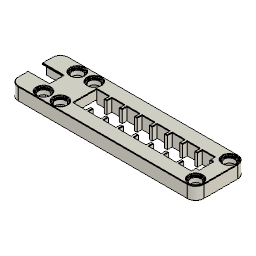
Mltplxr Chassis (Autodesk Fusion 360 design; units mm, degrees)
Autodesk Fusion 360 part; units mm, degrees
sketch "Skizze1" plane through (0, 0, 0) normal (0, 0, 1) x (1, 0, 0)
  line L0 (-39.6596, 9.8) -> (41.2404, 9.8)
  line L1 (41.2404, 9.8) -> (41.2404, -10.6)
  line L2 (41.2404, -10.6) -> (-39.6596, -10.6)
  line L3 (-39.6596, -10.6) -> (-39.6596, 9.8)
  line L4 (-39.6596, 4.85) -> (-29.1596, 4.85)
  line L5 (-29.1596, 4.85) -> (-29.1596, -5.65)
  line L6 (-29.1596, -5.65) -> (-39.6596, -5.65)
  line L7 (-39.6596, -5.65) -> (-39.6596, 4.85)
  line L8 (33.2404, 5.1) -> (39.0404, 5.1)
  line L9 (39.0404, 5.1) -> (39.0404, -5.9)
  line L10 (39.0404, -5.9) -> (33.2404, -5.9)
  line L11 (33.2404, -5.9) -> (33.2404, 5.1)
  line L12 (31.8975, 5.1) -> (31.8975, -5.9)
  line L13 (31.8975, -5.9) -> (26.0975, -5.9)
  line L14 (26.0975, 5.1) -> (31.8975, 5.1)
  line L15 (26.0975, -5.9) -> (26.0975, 5.1)
  line L16 (24.7547, 5.1) -> (24.7547, -5.9)
  line L17 (24.7547, -5.9) -> (18.9547, -5.9)
  line L18 (18.9547, 5.1) -> (24.7547, 5.1)
  line L19 (18.9547, -5.9) -> (18.9547, 5.1)
  line L20 (17.6118, 5.1) -> (17.6118, -5.9)
  line L21 (17.6118, -5.9) -> (11.8118, -5.9)
  line L22 (11.8118, 5.1) -> (17.6118, 5.1)
  line L23 (11.8118, -5.9) -> (11.8118, 5.1)
  line L24 (10.469, 5.1) -> (10.469, -5.9)
  line L25 (10.469, -5.9) -> (4.669, -5.9)
  line L26 (4.669, 5.1) -> (10.469, 5.1)
  line L27 (4.669, -5.9) -> (4.669, 5.1)
  line L28 (3.3261, 5.1) -> (3.3261, -5.9)
  line L29 (3.3261, -5.9) -> (-2.4739, -5.9)
  line L30 (-2.4739, 5.1) -> (3.3261, 5.1)
  line L31 (-2.4739, -5.9) -> (-2.4739, 5.1)
  line L32 (-3.8167, 5.1) -> (-3.8167, -5.9)
  line L33 (-3.8167, -5.9) -> (-9.6167, -5.9)
  line L34 (-9.6167, 5.1) -> (-3.8167, 5.1)
  line L35 (-9.6167, -5.9) -> (-9.6167, 5.1)
  line L36 (-10.9596, 5.1) -> (-10.9596, -5.9)
  line L37 (-10.9596, -5.9) -> (-16.7596, -5.9)
  line L38 (-16.7596, 5.1) -> (-10.9596, 5.1)
  line L39 (-16.7596, -5.9) -> (-16.7596, 5.1)
  line L40 (39.0404, 2.85) -> (40.5404, 2.85)
  line L41 (40.5404, 2.85) -> (40.5404, -3.65)
  line L42 (40.5404, -3.65) -> (39.0404, -3.65)
  line L43 (31.8975, 2.85) -> (33.3975, 2.85)
  line L44 (33.3975, -3.65) -> (31.8975, -3.65)
  line L45 (24.7547, 2.85) -> (26.2547, 2.85)
  line L46 (26.2547, -3.65) -> (24.7547, -3.65)
  line L47 (17.6118, 2.85) -> (19.1118, 2.85)
  line L48 (19.1118, -3.65) -> (17.6118, -3.65)
  line L49 (10.469, 2.85) -> (11.969, 2.85)
  line L50 (11.969, -3.65) -> (10.469, -3.65)
  line L51 (3.3261, 2.85) -> (4.8261, 2.85)
  line L52 (4.8261, -3.65) -> (3.3261, -3.65)
  line L53 (-3.8167, 2.85) -> (-2.3167, 2.85)
  line L54 (-2.3167, -3.65) -> (-3.8167, -3.65)
  line L55 (-10.9596, 2.85) -> (-9.4596, 2.85)
  line L56 (-9.4596, -3.65) -> (-10.9596, -3.65)
  line L57 (-39.6596, 2.85) -> (-30.2596, 2.85)
  line L58 (-30.2596, 2.85) -> (-30.2596, -3.65)
  line L59 (-30.2596, -3.65) -> (-39.6596, -3.65)
  arc A0 (-11.4096, 9.8) -> (-6.9096, 9.8) centre (-9.1596, 9.8) ccw
  arc A1 (-30.8596, 9.8) -> (-28.8596, 9.8) centre (-29.8596, 9.8) ccw
  arc A2 (9.0404, 9.8) -> (11.0404, 9.8) centre (10.0404, 9.8) ccw
  arc A3 (28.8404, 9.8) -> (32.8404, 9.8) centre (30.8404, 9.8) ccw
  line L60 (53, -0.4) -> (55.6063, -0.4)
  arc A4 (-28.8596, -10.6) -> (-30.8596, -10.6) centre (-29.8596, -10.6) ccw
  arc A5 (-6.9096, -10.6) -> (-11.4096, -10.6) centre (-9.1596, -10.6) ccw
  arc A6 (11.0404, -10.6) -> (9.0404, -10.6) centre (10.0404, -10.6) ccw
  arc A7 (32.8404, -10.6) -> (28.8404, -10.6) centre (30.8404, -10.6) ccw
  circle A8 centre (41.2404, -0.4) radius 1
  arc A9 (41.2404, -2.4) -> (41.2404, 1.6) centre (41.2404, -0.4) ccw
  line L61 (-29.1596, 8.8) -> (-16.7596, 8.8)
  line L62 (-16.7596, 8.8) -> (-16.7596, -9.6)
  line L63 (-16.7596, -9.6) -> (-29.1596, -9.6)
  line L64 (-29.1596, -9.6) -> (-29.1596, 8.8)
  dimension "d3" = -50
  dimension "d4" = 0
  dimension "d6" = 11
  dimension "d9" = 10.5
  dimension "d10" = 5.8
  dimension "d11" = 1.3429
  dimension "d71" = 6.5
  dimension "d72" = 2.25
  dimension "d73" = 2.25
  dimension "d88" = 6.5
  dimension "d89" = 9.4
  dimension "d93" = 10.5
  dimension "d112" = 2
  dimension "d113" = 4.5
  dimension "d116" = 2
  dimension "d120" = 4
  dimension "d128" = 20.4
  dimension "d130" = 10.2
  dimension "d131" = 20.4
  dimension "d132" = 20.4
  dimension "d133" = 20.4
  dimension "d134" = 20.4
  dimension "d135" = 4.7
  dimension "d136" = 4.7
  dimension "d146" = 4.95
  dimension "d147" = 4.95
  dimension "d148" = 6.95
  dimension "d149" = 6.95
  dimension "d151" = 1.5
  dimension "d152" = 2.2
  dimension "d198" = 4
  dimension "d199" = 2
  dimension "d204" = 1
  dimension "d205" = 1
  dimension "d214" = 9.8
  dimension "d229" = 80.9
  constraint horizontal L0
  constraint vertical L1
  constraint horizontal L2
  constraint vertical L3
  constraint horizontal L4
  constraint vertical L5
  constraint horizontal L6
  constraint vertical L7
  constraint horizontal L8
  constraint vertical L9
  constraint horizontal L10
  constraint vertical L11
  constraint coincident L9 L40.start
  constraint perpendicular L9 L40
  constraint perpendicular L40 L41
  constraint coincident L9 L42.end
  constraint perpendicular L9 L42
  constraint coincident L3 L57.start
  constraint coincident L7 L57.start
  constraint perpendicular L7 L57
  constraint perpendicular L56 L58
  constraint coincident L7 L59.end
  constraint coincident L0 A0.end
  constraint coincident L0 A0.start
  constraint coincident L0 A1.end
  constraint coincident L0 A1.start
  constraint coincident L0 A2.end
  constraint coincident L0 A2.start
  constraint coincident L0 A3.end
  constraint coincident L0 A3.start
  constraint perpendicular L1 L60
  constraint symmetric A0.end L60 A5.start
  constraint symmetric A0.start L60 A5.end
  constraint symmetric A0 L60 A5
  constraint symmetric A1.end L60 A4.start
  constraint symmetric A1.start L60 A4.end
  constraint symmetric A1 L60 A4
  constraint symmetric A2.end L60 A6.start
  constraint symmetric A2.start L60 A6.end
  constraint symmetric A2 L60 A6
  constraint symmetric A3.end L60 A7.start
  constraint symmetric A3.start L60 A7.end
  constraint symmetric A3 L60 A7
  constraint horizontal L59
  constraint midpoint L1 A8.centre
  constraint concentric A8 A9
  constraint coincident L1 A9.end
  constraint coincident L1 A9.start
  constraint horizontal L61
  constraint vertical L62
  constraint horizontal L63
  constraint vertical L64
  measures "d6" distance of L8 L10
  measures "d9" distance of L4 L6
  measures "d10" distance of L9 L11
  measures "d11" distance of L11 L12
  measures "d71" distance of L40.end L41.end
  measures "d72" distance of L8 L40
  measures "d73" distance of L10 L42
  measures "d88" distance of L57.end L58.end
  measures "d89" distance of L57.start L57.end
  measures "d93" distance of L4.start L4.end
  measures "d112" diameter of A1
  measures "d113" diameter of A0
  measures "d116" diameter of A2
  measures "d120" diameter of A3
  measures "d128" distance of L0 L2
  measures "d130" distance of L2 L60
  measures "d131" distance of L2 A1.centre
  measures "d132" distance of L2 A0.centre
  measures "d133" distance of L2 A2.centre
  measures "d134" distance of L2 A3.centre
  measures "d135" distance of L0 L18
  measures "d136" distance of L2 L13
  measures "d146" distance of L0 L4
  measures "d147" distance of L2 L6
  measures "d148" distance of L0 L57
  measures "d149" distance of L2 L59
  measures "d151" distance of L9 L41
  measures "d152" distance of L1 L9
  measures "d198" diameter of A9
  measures "d199" diameter of A8
  measures "d204" distance of L0 L61
  measures "d205" distance of L2 L63
  measures "d214" distance of L0.start A1.centre
  measures "d229" distance of L1.end L2.end
sketch "Skizze2" plane through (0, 0, 0) normal (0, 0, 1) x (1, 0, 0)
  line L0 (-36.4596, 11.6) -> (43.5404, 11.6)
  line L1 (47.5404, 7.6) -> (47.5404, -8.4)
  line L2 (43.5404, -12.4) -> (-36.4596, -12.4)
  line L3 (-40.4596, -8.4) -> (-40.4596, 7.6)
  line L4 (-39.6596, 9.8) -> (41.2404, 9.8)
  line L5 (41.2404, -10.6) -> (-39.6596, -10.6)
  line L6 (-39.6596, -10.6) -> (-39.6596, 9.8)
  line L7 (39.0404, 5.1) -> (39.0404, -5.9)
  line L8 (33.2404, -5.9) -> (33.2404, 5.1)
  line L9 (-27.8596, 4) -> (-27.8596, -4.8)
  line L10 (-29.9596, -4.8) -> (-27.8596, -4.8)
  line L11 (41.2404, 9.8) -> (41.2404, -10.6)
  line L12 (-39.6596, 4.85) -> (-40.4596, 4.85)
  line L13 (-39.6596, -5.65) -> (-40.4596, -5.65)
  line L14 (-39.6596, 2.85) -> (-30.2596, 2.85)
  line L15 (-30.2596, 2.85) -> (-30.2596, -3.65)
  line L16 (-30.2596, -3.65) -> (-39.6596, -3.65)
  line L17 (-39.6596, 2.85) -> (-40.4596, 2.85)
  line L18 (-39.6596, -3.65) -> (-40.4596, -3.65)
  arc A0 (47.5404, 7.6) -> (43.5404, 11.6) centre (43.5404, 7.6) ccw
  arc A1 (43.5404, -12.4) -> (47.5404, -8.4) centre (43.5404, -8.4) ccw
  line L19 (-16.7596, -5.9) -> (-16.7596, 5.1)
  arc A2 (-6.9096, -10.6) -> (-11.4096, -10.6) centre (-9.1596, -10.6) ccw
  arc A3 (-11.4096, 9.8) -> (-6.9096, 9.8) centre (-9.1596, 9.8) ccw
  arc A4 (28.8404, 9.8) -> (32.8404, 9.8) centre (30.8404, 9.8) ccw
  arc A5 (32.8404, -10.6) -> (28.8404, -10.6) centre (30.8404, -10.6) ccw
  circle A6 centre (-9.1596, 9.1) radius 2
  line L20 (-27.8596, 4) -> (-32, 4)
  line L21 (-32, 4) -> (-32, -4.8)
  line L22 (-29.9596, -4.8) -> (-32, -4.8)
  circle A7 centre (-9.1596, 9.1) radius 0.75
  line L23 (-15.2596, 4) -> (37.5404, 4)
  line L24 (37.5404, 4) -> (37.5404, -4.8)
  line L25 (37.5404, -4.8) -> (-15.2596, -4.8)
  line L26 (-15.2596, -4.8) -> (-15.2596, 4)
  line L27 (-29.1596, -5.65) -> (-39.6596, -5.65)
  line L28 (-39.6596, 4.85) -> (-29.1596, 4.85)
  circle A8 centre (-9.1596, 9.1) radius 1.25
  line L29 (-29.1596, -5.65) -> (-30.2596, -5.65)
  line L30 (-30.2596, -5.65) -> (-30.2596, 4.85)
  line L31 (-30.2596, 4.85) -> (-29.1596, 4.85)
  line L32 (-29.1596, 4.85) -> (-29.1596, -5.65)
  line L33 (53, -0.4) -> (55.6063, -0.4)
  circle A9 centre (30.8404, 9.1) radius 0.75
  circle A10 centre (30.8404, 9.1) radius 1.25
  circle A11 centre (30.8404, 9.1) radius 2
  circle A12 centre (-9.1596, -9.9) radius 1.25
  circle A13 centre (-9.1596, -9.9) radius 2
  circle A14 centre (-9.1596, -9.9) radius 0.75
  circle A15 centre (30.8404, -9.9) radius 2
  circle A16 centre (30.8404, -9.9) radius 1.25
  circle A17 centre (30.8404, -9.9) radius 0.75
  arc A18 (-36.4596, 11.6) -> (-40.4596, 7.6) centre (-36.4596, 7.6) ccw
  arc A19 (-40.4596, -8.4) -> (-36.4596, -12.4) centre (-36.4596, -8.4) ccw
  line L34 (-16.7596, -9.6) -> (-29.1596, -9.6)
  line L35 (-29.1596, -9.6) -> (-29.1596, 8.8)
  line L36 (-29.1596, 8.8) -> (-16.7596, 8.8)
  line L37 (-16.7596, 8.8) -> (-16.7596, -9.6)
  point P0 (-40.4596, 11.6)
  point P1 (47.5404, 11.6)
  point P2 (47.5404, -12.4)
  dimension "d16" = 24
  dimension "d17" = 88
  dimension "d18" = 1.8
  dimension "d19" = 1.8
  dimension "d20" = 0.8
  dimension "d122" = 4
  dimension "d123" = 4
  dimension "d124" = 4.95
  dimension "d125" = 4.95
  dimension "d143" = 6.95
  dimension "d144" = 6.95
  dimension "d150" = 10.2
  dimension "d154" = 2.25
  dimension "d162" = 4
  dimension "d167" = 1.5
  dimension "d171" = 8.8
  dimension "d172" = 8.8
  dimension "d173" = 1.5
  dimension "d174" = 1.5
  dimension "d175" = 5.8
  dimension "d176" = 5.8
  dimension "d179" = 2.5
  dimension "d200" = 1.1
  dimension "d218" = 40
  dimension "d219" = -8
  dimension "d220" = 5.8
  dimension "d230" = 4
  dimension "d231" = 2.5
  constraint horizontal L0
  constraint vertical L1
  constraint horizontal L2
  constraint vertical L3
  constraint vertical L9
  constraint perpendicular L9 L10
  constraint coincident L6 L12.start
  constraint coincident L3 L12.end
  constraint perpendicular L3 L12
  constraint coincident L6 L13.start
  constraint coincident L3 L13.end
  constraint perpendicular L3 L13
  constraint coincident L14.start L17.start
  constraint coincident L3 L17.end
  constraint perpendicular L3 L17
  constraint coincident L16.end L18.start
  constraint coincident L3 L18.end
  constraint perpendicular L3 L18
  constraint coincident P1 L0
  constraint coincident P1 L1
  constraint tangent L0 A0
  constraint tangent L1 A0
  constraint coincident P2 L1
  constraint coincident P2 L2
  constraint tangent L1 A1
  constraint tangent L2 A1
  constraint perpendicular L16 L21
  constraint perpendicular L21 L22
  constraint horizontal L23
  constraint vertical L24
  constraint horizontal L25
  constraint vertical L26
  constraint horizontal L29
  constraint vertical L30
  constraint horizontal L31
  constraint vertical L32
  constraint coincident L28 L30.end
  constraint coincident L27.start L29.start
  constraint symmetric A6 L33 A13
  constraint symmetric A7 L33 A14
  constraint symmetric A8 L33 A12
  constraint symmetric L33 A9 A17
  constraint symmetric L33 A10 A16
  constraint symmetric L33 A11 A15
  constraint coincident P0 L0
  constraint coincident P0 L3
  constraint tangent L0 A18
  constraint tangent L3 A18
  constraint tangent L2 A19
  constraint tangent L3 A19
  constraint equal A18 A19
  measures "d16" distance of P1 P2
  measures "d17" distance of P0 P1
  measures "d18" distance of L0 L4
  measures "d19" distance of L2 L5
  measures "d20" distance of L3 L6
  measures "d122" radius of A0
  measures "d123" radius of A1
  measures "d124" distance of L5 L13.start
  measures "d125" distance of L4 L12.start
  measures "d143" distance of L5 L18
  measures "d144" distance of L4 L17
  measures "d150" distance of L3 L15
  measures "d154" distance of L4 A3
  measures "d162" diameter of A6
  measures "d167" diameter of A7
  measures "d171" distance of L23.start L25.end
  measures "d172" distance of L9.start L9.end
  measures "d173" distance of L19 L26
  measures "d174" distance of L7 L24
  measures "d175" distance of L4 L23
  measures "d176" distance of L5 L25
  measures "d179" diameter of A8
  measures "d200" distance of L30 L32
  measures "d220" distance of L4 L20
  measures "d230" radius of A18
  measures "d231" distance of L0 A6.centre
sketch "Skizze3" plane through (0, 0, 0) normal (0, 0, 1) x (1, 0, 0)
  line L0 (43.5404, -12.4) -> (-36.4596, -12.4)
  line L1 (-40.4596, -8.4) -> (-40.4596, 7.6)
  line L2 (-36.4596, 11.6) -> (43.5404, 11.6)
  line L3 (47.5404, 7.6) -> (47.5404, -8.4)
  circle A0 centre (-36.4596, 7.6) radius 2.45
  circle A1 centre (-36.4596, 7.6) radius 3.25
  circle A2 centre (-28.4596, 7.6) radius 2.45
  circle A3 centre (-28.4596, 7.6) radius 3.25
  circle A4 centre (-20.4596, 7.6) radius 2.45
  circle A5 centre (-20.4596, 7.6) radius 3.25
  circle A6 centre (-12.4596, 7.6) radius 2.45
  circle A7 centre (-12.4596, 7.6) radius 3.25
  circle A8 centre (-4.4596, 7.6) radius 2.45
  circle A9 centre (-4.4596, 7.6) radius 3.25
  circle A10 centre (3.5404, 7.6) radius 2.45
  circle A11 centre (3.5404, 7.6) radius 3.25
  circle A12 centre (11.5404, 7.6) radius 2.45
  circle A13 centre (11.5404, 7.6) radius 3.25
  circle A14 centre (19.5404, 7.6) radius 2.45
  circle A15 centre (19.5404, 7.6) radius 3.25
  circle A16 centre (27.5404, 7.6) radius 2.45
  circle A17 centre (27.5404, 7.6) radius 3.25
  circle A18 centre (35.5404, 7.6) radius 2.45
  circle A19 centre (35.5404, 7.6) radius 3.25
  circle A20 centre (43.5404, 7.6) radius 2.45
  circle A21 centre (43.5404, 7.6) radius 3.25
  circle A22 centre (-36.4596, -0.4) radius 2.45
  circle A23 centre (-36.4596, -0.4) radius 3.25
  circle A24 centre (-28.4596, -0.4) radius 2.45
  circle A25 centre (-28.4596, -0.4) radius 3.25
  circle A26 centre (-20.4596, -0.4) radius 2.45
  circle A27 centre (-20.4596, -0.4) radius 3.25
  circle A28 centre (-12.4596, -0.4) radius 2.45
  circle A29 centre (-12.4596, -0.4) radius 3.25
  circle A30 centre (-4.4596, -0.4) radius 2.45
  circle A31 centre (-4.4596, -0.4) radius 3.25
  circle A32 centre (3.5404, -0.4) radius 2.45
  circle A33 centre (3.5404, -0.4) radius 3.25
  circle A34 centre (11.5404, -0.4) radius 2.45
  circle A35 centre (11.5404, -0.4) radius 3.25
  circle A36 centre (19.5404, -0.4) radius 2.45
  circle A37 centre (19.5404, -0.4) radius 3.25
  circle A38 centre (27.5404, -0.4) radius 2.45
  circle A39 centre (27.5404, -0.4) radius 3.25
  circle A40 centre (35.5404, -0.4) radius 2.45
  circle A41 centre (35.5404, -0.4) radius 3.25
  circle A42 centre (43.5404, -0.4) radius 2.45
  circle A43 centre (43.5404, -0.4) radius 3.25
  circle A44 centre (-36.4596, -8.4) radius 2.45
  circle A45 centre (-36.4596, -8.4) radius 3.25
  circle A46 centre (-28.4596, -8.4) radius 2.45
  circle A47 centre (-28.4596, -8.4) radius 3.25
  circle A48 centre (-20.4596, -8.4) radius 2.45
  circle A49 centre (-20.4596, -8.4) radius 3.25
  circle A50 centre (-12.4596, -8.4) radius 2.45
  circle A51 centre (-12.4596, -8.4) radius 3.25
  circle A52 centre (-4.4596, -8.4) radius 2.45
  circle A53 centre (-4.4596, -8.4) radius 3.25
  circle A54 centre (3.5404, -8.4) radius 2.45
  circle A55 centre (3.5404, -8.4) radius 3.25
  circle A56 centre (11.5404, -8.4) radius 2.45
  circle A57 centre (11.5404, -8.4) radius 3.25
  circle A58 centre (19.5404, -8.4) radius 2.45
  circle A59 centre (19.5404, -8.4) radius 3.25
  circle A60 centre (27.5404, -8.4) radius 2.45
  circle A61 centre (27.5404, -8.4) radius 3.25
  circle A62 centre (35.5404, -8.4) radius 2.45
  circle A63 centre (35.5404, -8.4) radius 3.25
  circle A64 centre (43.5404, -8.4) radius 2.45
  circle A65 centre (43.5404, -8.4) radius 3.25
  dimension "d34" = 4.9
  dimension "d35" = 6.5
  dimension "d36" = 4
  dimension "d37" = 4
  dimension "d40" = 80
  dimension "d41" = -16
  constraint concentric A0 A1
  measures "d34" diameter of A0
  measures "d35" diameter of A1
  measures "d36" distance of L1 A0.centre
  measures "d37" distance of L2 A0.centre
extrude "Platine - Extrusion (1)" add sketch "Skizze1" along normal blind 1.4 contours L0 L1 L3 L4 L8 L9 L11 L12 L14 L15 L16 L18 L19 L20 L22 L23 L24 L26 L27 L28 L30 L31 L32 L34 L35 L36 L38 L40 L41 L43 L45 L47 L49 L51 L53 L55 A0 A1 A2 A3 A8 L61 L62 L64 | L3 L4 L5 L6 L7 L57 L58 L59 L64 | L3 L7 L57 L58 L59 | L5 L39 L61 L62 L63 L64 | L1 L2 L3 L6 L9 L10 L11 L12 L13 L15 L16 L17 L19 L20 L21 L23 L24 L25 L27 L28 L29 L31 L32 L33 L35 L36 L37 L41 L42 L44 L46 L48 L50 L52 L54 L56 A4 A5 A6 A7 A8 L62 L63 L64 | L36 L37 L38 L39 L62 | L35 L36 L55 L56 | L32 L33 L34 L35 | L1 A8 A9 | L31 L32 L53 L54 | L9 L40 L41 L42 A8 | L28 L29 L30 L31 | L8 L9 L10 L11 | L27 L28 L51 L52 | L24 L25 L26 L27 | L11 L12 L43 L44 | L12 L13 L14 L15 | L23 L24 L49 L50 | L20 L21 L22 L23 | L15 L16 L45 L46 | L16 L17 L18 L19 | L19 L20 L47 L48 makes body 1
extrude "Platine - Extrusion (2)" add sketch "Skizze1" along normal blind 7 contours L3 L4 L5 L6 L7 L57 L58 L59 L64 | L3 L7 L57 L58 L59 bodies 1
extrude "Platine Extrusion (3)" add sketch "Skizze1" along normal blind 2.8 contours L5 L39 L61 L62 L63 L64 bodies 1
extrude "Platine Extrusion (4)" add sketch "Skizze1" along normal blind 10 contours L36 L37 L38 L39 L62 | L32 L33 L34 L35 | L28 L29 L30 L31 | L8 L9 L10 L11 | L24 L25 L26 L27 | L12 L13 L14 L15 | L20 L21 L22 L23 | L16 L17 L18 L19 bodies 1
extrude "Extrusion24" cut sketch "Skizze2" along normal blind 1 from surface at 6 contours L20 L28 L30 L31 L32 L35 | L10 L15 L20 L22 L30 L32 L35 | L10 L22 L27 L29 L30 L32 L35 bodies 1
extrude "Base" add sketch "Skizze2" against normal blind 4 separate body contours L0 L1 L2 L3 L4 L5 L6 L11 L12 L13 A0 A1 A6 A11 A13 A15 A18 A19 | L3 L6 L12 L17 | L3 L6 L17 L18 | L6 L14 L20 L21 L28 L30 | L4 L5 L6 L11 L19 A2 A3 A4 A5 A6 L27 L28 L29 L31 A11 A13 A15 L34 L35 L36 L37 | L3 L6 L13 L18 | L6 L14 L16 L21 | L20 L28 L30 L31 L32 L35 | L6 L16 L21 L22 L27 L30 | L14 L20 L21 L30 | L14 L15 L16 L21 L30 | L4 A3 A6 | L9 L10 L19 L20 L32 L34 L35 L36 L37 | L10 L15 L20 L22 L30 L32 L35 | L16 L21 L22 L30 | L4 A6 A8 | L4 A3 A6 A8 | A3 A6 | L9 L10 L20 L32 L35 | L10 L22 L27 L29 L30 L32 L35 | L4 A3 A6 | L5 A2 A13 | L5 A2 A12 A13 | L5 A12 A13 | A2 A13 | L4 A4 A11 | L5 A2 A13 | L4 A10 A11 | L4 A4 A10 A11 | A4 A11 | L4 A4 A11 | L5 A5 A15 | L5 A5 A15 A16 | L5 A15 A16 | A5 A15 | L5 A5 A15 | L8 L23 L25 L26 | L8 L23 L24 L25 makes body 2
extrude "Extrusion17" add sketch "Skizze2" along normal blind 1.8 contours L0 L1 L2 L3 L4 L5 L6 L11 L12 L13 A0 A1 A6 A11 A13 A15 A18 A19 | L3 L6 L12 L17 | L3 L6 L17 L18 | L3 L6 L13 L18 | L4 A6 A8 | L5 A12 A13 | L4 A10 A11 | L5 A15 A16 bodies 2
extrude "Base (1)" cut sketch "Skizze2" against normal blind 2 contours L14 L20 L21 L30 | L14 L15 L16 L21 L30 | L10 L15 L20 L22 L30 L32 L35 | L16 L21 L22 L30 | L9 L10 L20 L32 L35 | L8 L23 L25 L26 | L8 L23 L24 L25 bodies 2
extrude "Base - Löcher" cut sketch "Skizze3" against normal blind 5.8 from surface at 1.8 contours A0 | A2 | A4 | A10 | A12 | A14 | A20 | A22 | A26 | A42 | A44 | A46 | A48 | A54 | A56 | A58 | A64 bodies 2
extrude "Base - Ränder" cut sketch "Skizze3" along normal blind 0.9 from surface at -4 contours A1 | A3 | A5 | A11 | A13 | A15 | A21 | A23 | A27 | A43 | A45 | A47 | A49 | A55 | A57 | A59 | A65 bodies 2
extrude "Extrusion25" cut sketch "Skizze2" along normal blind 1.4 from surface at -4 contours L4 A6 A8 | L4 A3 A6 A8 | A3 A6 | L5 A2 A12 A13 | L5 A12 A13 | A2 A13 | L4 A10 A11 | L4 A4 A10 A11 | A4 A11 | L5 A5 A15 A16 | L5 A15 A16 | A5 A15 bodies 2
extrude "Base - Ränder2" cut sketch "Skizze3" against normal blind 2.7 from surface at 1.8 contours A1 | A3 | A5 | A11 | A13 | A15 | A21 | A23 | A27 | A43 | A45 | A47 | A49 | A55 | A57 | A59 | A65 bodies 2
extrude "Extrusion6" add sketch "Skizze3" sketch "Skizze2" sketch "Skizze1" along normal blind 1.8 from surface at 1.8 separate body contours A20 | A42 | A64 of sketch 2 contours L0 L1 L2 L3 L4 L5 L6 L11 L12 L13 A0 A1 A6 A11 A13 A15 A18 A19 | L4 A3 A6 | L4 A6 A8 | L4 A3 A6 A8 | L4 A7 A8 | L4 A7 A8 | L4 A3 A6 | L5 A2 A13 | L5 A2 A12 A13 | L5 A12 A13 | L4 A4 A11 | L5 A12 A14 | L5 A12 A14 | L5 A2 A13 | L4 A10 A11 | L4 A4 A10 A11 | L4 A9 A10 | L4 A9 A10 | L4 A4 A11 | L5 A5 A15 | L5 A5 A15 A16 | L5 A15 A16 | L5 A16 A17 | L5 A16 A17 | L5 A5 A15 | L5 A17 picked at (30.7858, -10.6106) of sketch 3 contours L0 L1 L3 L4 L8 L9 L11 L12 L14 L15 L16 L18 L19 L20 L22 L23 L24 L26 L27 L28 L30 L31 L32 L34 L35 L36 L38 L40 L41 L43 L45 L47 L49 L51 L53 L55 A0 A1 A2 A3 A8 L61 L62 L64 | L0 A1 | L1 L2 L3 L6 L9 L10 L11 L12 L13 L15 L16 L17 L19 L20 L21 L23 L24 L25 L27 L28 L29 L31 L32 L33 L35 L36 L37 L41 L42 L44 L46 L48 L50 L52 L54 L56 A4 A5 A6 A7 A8 L62 L63 L64 | L0 A2 | L2 A4 | L2 A6 | L1 L41 A8 makes body 3
extrude "Extrusion7" add sketch "Skizze2" sketch "Skizze1" along normal blind 3.7 from surface at 3.6 contours L0 L1 L2 L3 L4 L5 L6 L11 L12 L13 A0 A1 A6 A11 A13 A15 A18 A19 | L4 A3 A6 | L4 A6 A8 | L4 A3 A6 A8 | L4 A7 A8 | L4 A7 A8 | L4 A3 A6 | L5 A2 A13 | L5 A2 A12 A13 | L5 A12 A13 | L4 A4 A11 | L5 A12 A14 | L5 A12 A14 | L5 A2 A13 | L4 A10 A11 | L4 A4 A10 A11 | L4 A9 A10 | L4 A9 A10 | L4 A4 A11 | L5 A5 A15 | L5 A5 A15 A16 | L5 A15 A16 | L5 A16 A17 | L5 A16 A17 | L5 A5 A15 of sketch 2 contours L0 L1 L3 L4 L8 L9 L11 L12 L14 L15 L16 L18 L19 L20 L22 L23 L24 L26 L27 L28 L30 L31 L32 L34 L35 L36 L38 L40 L41 L43 L45 L47 L49 L51 L53 L55 A0 A1 A2 A3 A8 L61 L62 L64 | L0 A1 | L5 L39 L61 L62 L63 L64 | L1 L2 L3 L6 L9 L10 L11 L12 L13 L15 L16 L17 L19 L20 L21 L23 L24 L25 L27 L28 L29 L31 L32 L33 L35 L36 L37 L41 L42 L44 L46 L48 L50 L52 L54 L56 A4 A5 A6 A7 A8 L62 L63 L64 | L0 A2 | L2 A4 | L2 A6 bodies 3
extrude "Extrusion8" add sketch "Skizze2" sketch "Skizze1" along normal blind 0.8 from surface at 7.2 contours L0 L1 L2 L3 L4 L5 L6 L11 L12 L13 A0 A1 A6 A11 A13 A15 A18 A19 | L3 L6 L12 L17 | L3 L6 L13 L18 | L4 A6 A8 | L4 A7 A8 | L4 A7 | L4 A7 | L5 A12 A13 | L5 A12 A14 | L4 A10 A11 | L5 A14 | L5 A14 | L4 A9 A10 | L4 A9 | L4 A9 | L5 A15 A16 | L5 A16 A17 | L5 A17 | L5 A17 picked at (-9.2359, 10.1786) picked at (-9.2359, -10.9786) picked at (30.9167, 10.1786) picked at (30.7641, -10.9786) of sketch 2 contours L0 L1 L3 L4 L8 L9 L11 L12 L14 L15 L16 L18 L19 L20 L22 L23 L24 L26 L27 L28 L30 L31 L32 L34 L35 L36 L38 L40 L41 L43 L45 L47 L49 L51 L53 L55 A0 A1 A2 A3 A8 L61 L62 L64 | L0 A1 | L3 L4 L5 L6 L7 L57 L58 L59 L64 | L5 L39 L61 L62 L63 L64 | L0 A0 | L1 L2 L3 L6 L9 L10 L11 L12 L13 L15 L16 L17 L19 L20 L21 L23 L24 L25 L27 L28 L29 L31 L32 L33 L35 L36 L37 L41 L42 L44 L46 L48 L50 L52 L54 L56 A4 A5 A6 A7 A8 L62 L63 L64 | L0 A2 | L2 A4 | L0 A3 | L2 A5 | L2 A6 | L1 L41 A8 | L2 A7 bodies 3
extrude "Case - Löcher tief" cut sketch "Skizze3" along normal blind 8 contours A2 | A4 | A20 | A46 | A48 | A64 bodies 3
extrude "Extrusion23" add sketch "Skizze2" along normal blind 0.5 from surface at 6.7 contours L20 L28 L30 L31 L32 L35 | L10 L15 L20 L22 L30 L32 L35 | L10 L22 L27 L29 L30 L32 L35 bodies 3
extrude "Case - Ränder2" cut sketch "Skizze3" against normal blind 0.9 from surface at 8 contours A3 | A5 | A21 | A47 | A49 | A65 bodies 3
extrude "Case - Ränder3" cut sketch "Skizze3" along normal blind 3 from surface at 1.8 contours A3 | A5 | A21 | A47 | A49 | A65 bodies 3
fillet "Abrundung2" radius 0.2 41 edges at (-31.4897, -7.2247, -0.9) (-23.4897, -7.2247, -0.9) (-23.4897, 0.7753, -0.9) (-23.4897, 8.7753, -0.9) (-39.4897, -7.2247, -0.9) (-39.4897, 8.7753, -0.9) (-39.4897, 0.7753, -0.9) (-31.4897, 8.7753, -0.9) (0.5103, 8.7753, -0.9) (0.5103, -7.2247, -0.9) (8.5103, -7.2247, -0.9) (8.5103, 8.7753, -0.9) (16.5103, 8.7753, -0.9) (16.5103, -7.2247, -0.9) (40.5103, 8.7753, -0.9) (40.5103, 0.7753, -0.9) (40.5103, -7.2247, -0.9) (-40.4596, -0.4, -4) (-39.288, 10.4284, -4) (3.5404, 11.6, -4) (46.3688, 10.4284, -4) (47.5404, -0.4, -4) (46.3688, -11.2284, -4) (3.5404, -12.4, -4) (-39.288, -11.2284, -4) (16.5103, 6.4247, -4) (8.5103, 6.4247, -4) (16.5103, -9.5753, -4) (8.5103, -9.5753, -4) (0.5103, 6.4247, -4) (0.5103, -9.5753, -4) (40.5103, -1.5753, -4) (40.5103, -9.5753, -4) (40.5103, 6.4247, -4) (-23.4897, -1.5753, -4) (-23.4897, 6.4247, -4) (-23.4897, -9.5753, -4) (-31.4897, -9.5753, -4) (-39.4897, -9.5753, -4) (-39.4897, -1.5753, -4) (-39.4897, 6.4247, -4) 17 faces at (-17.4975, 7.3168, -3.1) (-33.4975, -8.6832, -3.1) (46.5025, -8.6832, -3.1) (-17.4975, -0.6832, -3.1) (-17.4975, -8.6832, -3.1) (46.5025, -0.6832, -3.1) (-25.4975, -8.6832, -3.1) (14.5025, 7.3168, -3.1) (46.5025, 7.3168, -3.1) (-33.4975, -0.6832, -3.1) (22.5025, -8.6832, -3.1) (6.5116, -8.5615, -3.1) (6.5025, 7.3168, -3.1) (22.5025, 7.3168, -3.1) (-33.4975, 7.3168, -3.1) (14.5116, -8.5615, -3.1) (-25.4975, 7.3168, -3.1) on bodies 2
fillet "Abrundung3" radius 0.2 20 edges at (-30.2596, -0.4, 6.7) (-29.1596, -0.4, 6.7) (-35.3596, -3.65, 7.2) (-35.3596, -5.65, 7.2) (-35.3596, 4.85, 7.2) (-30.2596, -4.65, 7.2) (-30.2596, 3.85, 7.2) (-30.2596, -3.65, 7.6) (-35.3596, 2.85, 7.2) (-30.2596, 2.85, 7.6) (-40.4596, 4.85, 4.5) (-40.4596, -5.65, 4.5) (-40.4596, -4.65, 7.2) (-40.4596, 3.85, 7.2) (-40.4596, 2.85, 7.6) (-40.4596, -3.65, 7.6) (-29.7096, 4.85, 6.7) (-30.2596, 4.85, 6.95) (-30.2596, -5.65, 6.95) (-29.7096, -5.65, 6.7) 8 faces at (11.579, -9.9084, 8) (46.5025, 7.3168, 7.1) (46.5025, -8.6832, 7.1) (10.7166, 8.2342, 1.8) (-17.4975, 7.3168, 7.1) (-25.4975, 7.3168, 7.1) (-17.4975, -8.6832, 7.1) (-25.4975, -8.6832, 7.1) on bodies 3
extrude "Extrusion26" add sketch "Skizze3" sketch "Skizze1" along normal blind 0.4 from surface at 2.9 separate body contours A2 | A3 | A4 | A5 | A46 | A47 | A48 | A49 of sketch 2 contours L5 L39 L61 L62 L63 L64 makes body 4
move_face "Flächen versetzen1" offset -0.3 10 faces at (-16.7596, -3.4667, 3.1667) (-17.2127, 8.8, 3.1667) (-19.3518, 10.6554, 3.1667) (-24.7862, 8.8, 3.0333) (-30.7172, 9.9379, 3.0333) (-27.1689, -11.3827, 3.1667) (-29.1596, 1.2088, 3.1667) (-24.1331, -9.6, 3.1667) (-19.6604, -11.5502, 3.1667) (-16.9862, -9.6, 3.0333) on bodies 4
hidden bodies 1 2 4
equation "d124 = d125"
equation "d131 = d128"
equation "d132 = d128"
equation "d133 = d128"
equation "d134 = d128"
equation "d171 = d172"
equation "d174 = d173"
named bodies: "Mltplxr Platine", "Mltplxr Base", "Mltplxr Protector", "Mltplxr Case"
